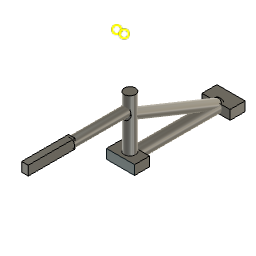
3d_1 (Autodesk Fusion 360 design; units mm, degrees)
Autodesk Fusion 360 part; units mm, degrees
cylinder "CylinderPrimitive1" add diameter 6 height 50 placed x (1, 0, 0) y (0, 0, -1) z (0, 1, 0) at (0, 0, 0) makes body 1
box "BoxPrimitive1" add length 8 width 15 height 5 placed x (0, 1, 0) y (-1, 0, 0) z (0, 0, 1) at (-5, 0, 0) separate body makes body 2
move_body "Move1" bodies 2 to x (1, 0, 0) y (0, 1, 0) z (0, 0, 1) at (12.5, 0, 0)
move_body "Move2" bodies 2 to x (1, 0, 0) y (0, 1, 0) z (0, 0, 1) at (0, 0, -2.7)
copy_body "CopyPasteBodies1" bodies 2 makes body 3
move_body "Move3" bodies 3 to x (1, 0, 0) y (0, 1, 0) z (0, 0, 1) at (0, 43, 0)
move_body "Move4" bodies 3 to x (1, 0, 0) y (0, 1, 0) z (0, 0, 1) at (0, 5, 0)
move_body "Move5" bodies 2 to x (1, 0, 0) y (0, 1, 0) z (0, 0, 1) at (0, -3, 0)
sketch "Sketch3" plane through (0, -3, 0) normal (0, -1, 0) x (1, 0, 0)
  line L0 (-7.5, 2.3) -> (-7.5, -2.7)
  line L1 (-7.5, -2.7) -> (7.5, -2.7)
  line L2 (7.5, -2.7) -> (7.5, 2.3)
  line L3 (7.5, 2.3) -> (-7.5, 2.3)
sketch "Sketch4" plane through (0, 0, 0) normal (1, 0, 0) x (0, 1, 0)
  line L0 (8.5, 0) -> (-3, 0)
  line L1 (-3, 0) -> (-3, 60.0139)
  line L2 (-3, 60.0139) -> (8.5, 60.0139)
  line L3 (8.5, 60.0139) -> (8.5, 0)
  constraint horizontal L0
  constraint vertical L1
  constraint horizontal L2
cylinder "CylinderPrimitive2" add diameter 4.991 height 52 placed x (1, 0, 0) y (0, 0, -1) z (0, 1, 0) at (0, 0, 35) separate body makes body 4
move_body "Move7" bodies 4 to x (1, 0, 0) y (0, 0.707107, -0.707107) z (0, 0.707107, 0.707107) at (0, -43.3149, 15.4563)
move_body "Move8" bodies 4 to x (1, 0, 0) y (0, 1, 0) z (0, 0, 1) at (0, 25, -7)
move_body "Move9" bodies 4 to x (1, 0, 0) y (0, 1, 0) z (0, 0, 1) at (0, -3.5355, 3.5355)
move_body "Move10" bodies 4 to x (1, 0, 0) y (0, 1, 0) z (0, 0, 1) at (0, 3, 5)
sketch "Sketch7" plane through (0, -3, 0) normal (0, -1, 0) x (1, 0, 0)
  line L0 (-2, 60.0139) -> (-2, 0)
  line L1 (-2, 0) -> (2, 0)
  line L2 (2, 0) -> (2, 60.0139)
sketch "Sketch8" plane through (0, 0, 0) normal (1, 0, 0) x (0, 1, 0)
  line L0 (-2.8843, 58.2072) -> (8.4016, 58.2072)
  line L1 (8.4016, 58.2072) -> (8.4016, 74.8756)
  line L2 (8.4016, 74.8756) -> (-2.8843, 74.8756)
  line L3 (-2.8843, 74.8756) -> (-2.8843, 58.2072)
  constraint horizontal L0
  constraint vertical L1
  constraint horizontal L2
  constraint vertical L3
cylinder "CylinderPrimitive3" add diameter 6 height 30 placed x (1, 0, 0) y (0, 1, 0) z (0, 0, 1) at (0, 2, 0) separate body makes body 5
move_body "Move12" bodies 4 to x (1, 0, 0) y (0, 1, 0) z (0, 0, 1) at (0, -3.5355, 3.5355)
move_body "Move13" bodies 4 to x (1, 0, 0) y (0, 1, 0) z (0, 0, 1) at (0, -3.5355, 3.5355)
move_body "Move14" bodies 4 to x (1, 0, 0) y (0, 0.996195, -0.087156) z (0, 0.087156, 0.996195) at (0, -0.0178, 4.1922)
move_body "Move15" bodies 4 to x (1, 0, 0) y (0, 1, 0) z (0, 0, 1) at (0, -1.9284, 2.2981)
move_body "Move17" bodies 4 to x (1, 0, 0) y (0, 1, 0) z (0, 0, 1) at (0, 3.8567, -4.5963)
move_body "Move18" bodies 4 to x (1, 0, 0) y (0, 1, 0) z (0, 0, 1) at (0, -0.6428, 0.766)
extrude "Extrude3" cut 1 faces at (-0.4454, 0.9948, 0) along direction (0, 0, 1) blind 2.1 on bodies 5 bodies 1 5
sketch "Sketch15" plane through (0, 0, 0) normal (1, 0, 0) x (0, 1, 0)
sketch "Sketch17" plane through (0, 0, 0) normal (0, 1, 0) x (1, 0, 0)
cylinder "CylinderPrimitive4" add diameter 5 height -30 placed x (1, 0, 0) y (0, 0, -1) z (0, 1, 0) at (0, 0, 22) separate body makes body 6
box "BoxPrimitive2" add length 5 width 3.5 height -25 placed x (0, 0, -1) y (-1, 0, 0) z (0, 1, 0) at (2.2492, 0, 24.1598) separate body makes body 7
move_body "Move19" bodies 7 to x (1, 0, 0) y (0, 1, 0) z (0, 0, 1) at (-0.5, -5, 0.5)
move_body "Move20" bodies 7 to x (1, 0, 0) y (0, 1, 0) z (0, 0, 1) at (0, -25, 0)
move_body "Move21" bodies 7 to x (1, 0, 0) y (0, 1, 0) z (0, 0, 1) at (0, 1, 0)
move_body "Move22" bodies 4 to x (1, 0, 0) y (0, 0.939693, 0.34202) z (0, -0.34202, 0.939693) at (0, 23.0375, 1.0993)
move_body "Move23" bodies 4 to x (1, 0, 0) y (0, 1, 0) z (0, 0, 1) at (0, -10, -30)
move_body "Move24" bodies 4 to x (1, 0, 0) y (0, 0.996195, 0.087156) z (0, -0.087156, 0.996195) at (0, 0.3831, -4.1747)
move_body "Move25" bodies 4 to x (1, 0, 0) y (0, 1, 0) z (0, 0, 1) at (0, 0, 5)
move_body "Move26" bodies 4 to x (1, 0, 0) y (0, 1, 0) z (0, 0, 1) at (0, 1.8126, -0.8452)
move_body "Move27" bodies 4 to x (1, 0, 0) y (0, 0.996195, 0.087156) z (0, -0.087156, 0.996195) at (0, 0.4136, -4.872)
move_body "Move28" bodies 4 to x (1, 0, 0) y (0, 1, 0) z (0, 0, 1) at (0, 0, 3)
move_body "Move29" bodies 4 to x (1, 0, 0) y (0, 0.999391, -0.034899) z (0, 0.034899, 0.999391) at (0, -0.0462, 1.9558)
move_body "Move30" bodies 4 to x (1, 0, 0) y (0, 1, 0) z (0, 0, 1) at (0, 0.9272, -0.3746)
